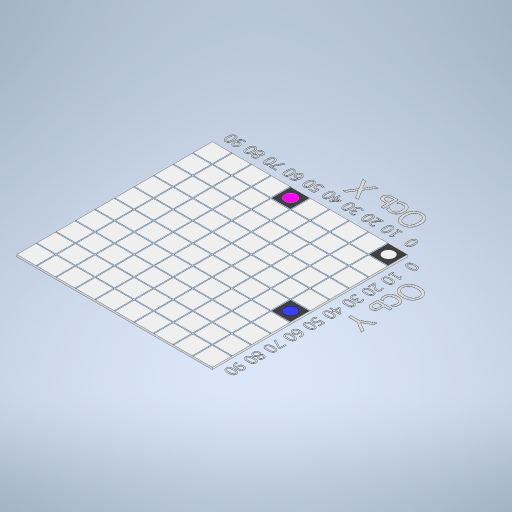
# Autodesk Inventor part: поле
Saved by Autodesk Inventor 2023.2 (Build 272271030, 271C)
## iProperties
Created: 2025-05-13
Part Number: поле
Material: Типовые
Document SubType Name: Modeling
Designer: e5470
Density: 1 g/cm^3
Appearance: По умолчанию
Author: e5470
Autodesk Inventor part; units mm, degrees
(part 1 of 3)
ref_plane "YZ Plane" through (0, 0, 0) normal (1, 0, 0) x (0, 1, 0)
ref_plane "XZ Plane" through (0, 0, 0) normal (0, 1, 0) x (-1, 0, 0)
ref_plane "XY Plane" through (0, 0, 0) normal (0, 0, 1) x (1, 0, 0)
sketch "Эскиз1" plane through (0, 0, 0) normal (0, 1, 0) x (-1, 0, 0)
  line L0 (-500, -500) -> (500, -500)
  line L1 (500, -500) -> (500, 500)
  line L2 (500, 500) -> (-500, 500)
  line L3 (-500, 500) -> (-500, -500)
  line L4 (-500, -500) -> (500, 500) construction
  line L5 (500, -500) -> (-500, 500) construction
  point P0 (0, 0)
  dimension "d0" = 1000
  dimension "d1" = 1000
  constraints: 12 end point, 2 midpoint, 2 parallel, 1 horizontal, 1 perpendicular
  measures "d0" distance of L2.end L1.end
  measures "d1" distance of L1.end L0.end
extrude "Выдавливание1" add sketch "Эскиз1" along normal blind 10
sketch "Эскиз2" plane through (0, 10, 0) normal (0, 1, 0) x (1, 0, 0)
  line L0 (500, -500) -> (500, 500) projected
  line L1 (-500, -2.5) -> (500, -2.5)
  line L2 (500, -2.5) -> (500, 2.5)
  line L3 (500, 2.5) -> (-500, 2.5)
  line L4 (-500, 2.5) -> (-500, -2.5)
  line L5 (-500, -2.5) -> (500, 2.5) construction
  line L6 (500, -2.5) -> (-500, 2.5) construction
  line L7 (-500, 97.5) -> (500, 97.5)
  line L8 (500, 97.5) -> (500, 102.5)
  line L9 (500, 102.5) -> (-500, 102.5)
  line L10 (-500, 102.5) -> (-500, 97.5)
  line L11 (-500, 97.5) -> (500, 102.5) construction
  line L12 (500, 97.5) -> (-500, 102.5) construction
  line L13 (-500, 197.5) -> (500, 197.5)
  line L14 (500, 197.5) -> (500, 202.5)
  line L15 (500, 202.5) -> (-500, 202.5)
  line L16 (-500, 202.5) -> (-500, 197.5)
  line L17 (-500, 197.5) -> (500, 202.5) construction
  line L18 (500, 197.5) -> (-500, 202.5) construction
  line L19 (-500, 297.5) -> (500, 297.5)
  line L20 (500, 297.5) -> (500, 302.5)
  line L21 (500, 302.5) -> (-500, 302.5)
  line L22 (-500, 302.5) -> (-500, 297.5)
  line L23 (-500, 297.5) -> (500, 302.5) construction
  line L24 (500, 297.5) -> (-500, 302.5) construction
  line L25 (-500, 397.5) -> (500, 397.5)
  line L26 (500, 397.5) -> (500, 402.5)
  line L27 (500, 402.5) -> (-500, 402.5)
  line L28 (-500, 402.5) -> (-500, 397.5)
  line L29 (-500, 397.5) -> (500, 402.5) construction
  line L30 (500, 397.5) -> (-500, 402.5) construction
  line L31 (-500, -102.5) -> (500, -102.5)
  line L32 (500, -102.5) -> (500, -97.5)
  line L33 (500, -97.5) -> (-500, -97.5)
  line L34 (-500, -97.5) -> (-500, -102.5)
  line L35 (-500, -102.5) -> (500, -97.5) construction
  line L36 (500, -102.5) -> (-500, -97.5) construction
  line L37 (-500, -2.5) -> (500, -2.5)
  line L38 (500, -2.5) -> (500, 2.5)
  line L39 (500, 2.5) -> (-500, 2.5)
  line L40 (-500, 2.5) -> (-500, -2.5)
  line L41 (-500, -2.5) -> (500, 2.5) construction
  line L42 (500, -2.5) -> (-500, 2.5) construction
  line L43 (-500, 97.5) -> (500, 97.5)
  line L44 (500, 97.5) -> (500, 102.5)
  line L45 (500, 102.5) -> (-500, 102.5)
  line L46 (-500, 102.5) -> (-500, 97.5)
  line L47 (-500, 97.5) -> (500, 102.5) construction
  line L48 (500, 97.5) -> (-500, 102.5) construction
  line L49 (-500, 197.5) -> (500, 197.5)
  line L50 (500, 197.5) -> (500, 202.5)
  line L51 (500, 202.5) -> (-500, 202.5)
  line L52 (-500, 202.5) -> (-500, 197.5)
  line L53 (-500, 197.5) -> (500, 202.5) construction
  line L54 (500, 197.5) -> (-500, 202.5) construction
  line L55 (-500, 297.5) -> (500, 297.5)
  line L56 (500, 297.5) -> (500, 302.5)
  line L57 (500, 302.5) -> (-500, 302.5)
  line L58 (-500, 302.5) -> (-500, 297.5)
  line L59 (-500, 297.5) -> (500, 302.5) construction
  line L60 (500, 297.5) -> (-500, 302.5) construction
  line L61 (-500, -202.5) -> (500, -202.5)
  line L62 (500, -202.5) -> (500, -197.5)
  line L63 (500, -197.5) -> (-500, -197.5)
  line L64 (-500, -197.5) -> (-500, -202.5)
  line L65 (-500, -202.5) -> (500, -197.5) construction
  line L66 (500, -202.5) -> (-500, -197.5) construction
  line L67 (-500, -102.5) -> (500, -102.5)
  line L68 (500, -102.5) -> (500, -97.5)
  line L69 (500, -97.5) -> (-500, -97.5)
  line L70 (-500, -97.5) -> (-500, -102.5)
  line L71 (-500, -102.5) -> (500, -97.5) construction
  line L72 (500, -102.5) -> (-500, -97.5) construction
  line L73 (-500, -2.5) -> (500, -2.5)
  line L74 (500, -2.5) -> (500, 2.5)
  line L75 (500, 2.5) -> (-500, 2.5)
  line L76 (-500, 2.5) -> (-500, -2.5)
  line L77 (-500, -2.5) -> (500, 2.5) construction
  line L78 (500, -2.5) -> (-500, 2.5) construction
  line L79 (-500, 97.5) -> (500, 97.5)
  line L80 (500, 97.5) -> (500, 102.5)
  line L81 (500, 102.5) -> (-500, 102.5)
  line L82 (-500, 102.5) -> (-500, 97.5)
  line L83 (-500, 97.5) -> (500, 102.5) construction
  line L84 (500, 97.5) -> (-500, 102.5) construction
  line L85 (-500, 197.5) -> (500, 197.5)
  line L86 (500, 197.5) -> (500, 202.5)
  line L87 (500, 202.5) -> (-500, 202.5)
  line L88 (-500, 202.5) -> (-500, 197.5)
  line L89 (-500, 197.5) -> (500, 202.5) construction
  line L90 (500, 197.5) -> (-500, 202.5) construction
  line L91 (-500, -302.5) -> (500, -302.5)
  line L92 (500, -302.5) -> (500, -297.5)
  line L93 (500, -297.5) -> (-500, -297.5)
  line L94 (-500, -297.5) -> (-500, -302.5)
  line L95 (-500, -302.5) -> (500, -297.5) construction
  line L96 (500, -302.5) -> (-500, -297.5) construction
  line L97 (-500, -202.5) -> (500, -202.5)
  line L98 (500, -202.5) -> (500, -197.5)
  line L99 (500, -197.5) -> (-500, -197.5)
  line L100 (-500, -197.5) -> (-500, -202.5)
  line L101 (-500, -202.5) -> (500, -197.5) construction
  line L102 (500, -202.5) -> (-500, -197.5) construction
  line L103 (-500, -102.5) -> (500, -102.5)
  line L104 (500, -102.5) -> (500, -97.5)
  line L105 (500, -97.5) -> (-500, -97.5)
  line L106 (-500, -97.5) -> (-500, -102.5)
  line L107 (-500, -102.5) -> (500, -97.5) construction
  line L108 (500, -102.5) -> (-500, -97.5) construction
  line L109 (-500, -2.5) -> (500, -2.5)
  line L110 (500, -2.5) -> (500, 2.5)
  line L111 (500, 2.5) -> (-500, 2.5)
  line L112 (-500, 2.5) -> (-500, -2.5)
  line L113 (-500, -2.5) -> (500, 2.5) construction
  line L114 (500, -2.5) -> (-500, 2.5) construction
  line L115 (-500, 97.5) -> (500, 97.5)
  line L116 (500, 97.5) -> (500, 102.5)
  line L117 (500, 102.5) -> (-500, 102.5)
  line L118 (-500, 102.5) -> (-500, 97.5)
  line L119 (-500, 97.5) -> (500, 102.5) construction
  line L120 (500, 97.5) -> (-500, 102.5) construction
  line L121 (-500, -402.5) -> (500, -402.5)
  line L122 (500, -402.5) -> (500, -397.5)
  line L123 (500, -397.5) -> (-500, -397.5)
  line L124 (-500, -397.5) -> (-500, -402.5)
  line L125 (-500, -402.5) -> (500, -397.5) construction
  line L126 (500, -402.5) -> (-500, -397.5) construction
  line L127 (-500, -302.5) -> (500, -302.5)
  line L128 (500, -302.5) -> (500, -297.5)
  line L129 (500, -297.5) -> (-500, -297.5)
  line L130 (-500, -297.5) -> (-500, -302.5)
  line L131 (-500, -302.5) -> (500, -297.5) construction
  line L132 (500, -302.5) -> (-500, -297.5) construction
  line L133 (-500, -202.5) -> (500, -202.5)
  line L134 (500, -202.5) -> (500, -197.5)
  line L135 (500, -197.5) -> (-500, -197.5)
  line L136 (-500, -197.5) -> (-500, -202.5)
  line L137 (-500, -202.5) -> (500, -197.5) construction
  line L138 (500, -202.5) -> (-500, -197.5) construction
  line L139 (-500, -102.5) -> (500, -102.5)
  line L140 (500, -102.5) -> (500, -97.5)
  line L141 (500, -97.5) -> (-500, -97.5)
  line L142 (-500, -97.5) -> (-500, -102.5)
  line L143 (-500, -102.5) -> (500, -97.5) construction
  line L144 (500, -102.5) -> (-500, -97.5) construction
  line L145 (-500, -2.5) -> (500, -2.5)
  line L146 (500, -2.5) -> (500, 2.5)
  line L147 (500, 2.5) -> (-500, 2.5)
  line L148 (-500, 2.5) -> (-500, -2.5)
  line L149 (-500, -2.5) -> (500, 2.5) construction
  line L150 (500, -2.5) -> (-500, 2.5) construction
  line L151 (2.5, 500) -> (-2.5, 500)
  line L152 (2.5, 500) -> (-2.5, 500)
  line L153 (2.5, 500) -> (-2.5, 500)
  line L154 (-97.5, -500) -> (-97.5, 500)
  line L155 (-97.5, 500) -> (-102.5, 500)
  line L156 (-102.5, 500) -> (-102.5, -500)
  line L157 (-102.5, -500) -> (-97.5, -500)
  line L158 (-97.5, -500) -> (-102.5, 500) construction
  line L159 (-97.5, 500) -> (-102.5, -500) construction
  line L160 (-97.5, -500) -> (-97.5, 500)
  line L161 (-97.5, -500) -> (-97.5, 500)
  line L162 (-97.5, -500) -> (-97.5, 500)
  line L163 (-97.5, -500) -> (-102.5, 500) construction
  line L164 (-97.5, 500) -> (-102.5, -500) construction
  line L165 (-97.5, -500) -> (-102.5, 500) construction
  line L166 (-97.5, 500) -> (-102.5, -500) construction
  line L167 (-97.5, -500) -> (-102.5, 500) construction
  line L168 (-97.5, 500) -> (-102.5, -500) construction
  line L169 (-102.5, 500) -> (-102.5, -500)
  line L170 (-102.5, 500) -> (-102.5, -500)
  line L171 (-102.5, 500) -> (-102.5, -500)
  line L172 (-102.5, -500) -> (-97.5, -500)
  line L173 (-102.5, -500) -> (-97.5, -500)
  line L174 (-102.5, -500) -> (-97.5, -500)
  line L175 (-297.5, -500) -> (-297.5, 500)
  line L176 (-297.5, -500) -> (-297.5, 500)
  line L177 (-297.5, 500) -> (-302.5, 500)
  line L178 (-302.5, 500) -> (-302.5, -500)
  line L179 (-297.5, -500) -> (-302.5, 500) construction
  line L180 (-302.5, 500) -> (-302.5, -500)
  line L181 (-297.5, -500) -> (-302.5, 500) construction
  line L182 (-297.5, 500) -> (-302.5, -500) construction
  line L183 (-397.5, -500) -> (-397.5, 500)
  line L184 (-402.5, 500) -> (-402.5, -500)
  line L185 (-397.5, 500) -> (-402.5, -500) construction
  line L186 (-397.5, -500) -> (-402.5, 500) construction
  line L187 (-397.5, 500) -> (-402.5, 500)
  line L188 (-297.5, 500) -> (-302.5, -500) construction
  line L189 (-302.5, -500) -> (-297.5, -500)
  line L190 (-302.5, -500) -> (-297.5, -500)
  line L191 (-402.5, -500) -> (-397.5, -500)
  line L192 (-197.5, -500) -> (-197.5, 500)
  line L193 (-197.5, 500) -> (-202.5, 500)
  line L194 (-202.5, 500) -> (-202.5, -500)
  line L195 (-202.5, -500) -> (-197.5, -500)
  line L196 (-197.5, -500) -> (-202.5, 500) construction
  line L197 (-197.5, 500) -> (-202.5, -500) construction
  line L198 (-202.5, 500) -> (-202.5, -500)
  line L199 (-202.5, 500) -> (-202.5, -500)
  line L200 (-197.5, 500) -> (-202.5, -500) construction
  line L201 (-197.5, 500) -> (-202.5, -500) construction
  line L202 (-197.5, -500) -> (-202.5, 500) construction
  line L203 (-197.5, -500) -> (-202.5, 500) construction
  line L204 (-197.5, 500) -> (-202.5, 500)
  line L205 (-197.5, 500) -> (-202.5, 500)
  line L206 (-197.5, -500) -> (-197.5, 500)
  line L207 (-197.5, -500) -> (-197.5, 500)
  line L208 (-202.5, -500) -> (-197.5, -500)
  line L209 (-202.5, -500) -> (-197.5, -500)
  line L210 (-97.5, 500) -> (-102.5, 500)
  line L211 (-97.5, 500) -> (-102.5, 500)
  line L212 (-97.5, 500) -> (-102.5, 500)
  line L213 (202.5, -500) -> (202.5, 500)
  line L214 (202.5, 500) -> (197.5, 500)
  line L215 (197.5, 500) -> (197.5, -500)
  line L216 (197.5, -500) -> (202.5, -500)
  line L217 (202.5, -500) -> (197.5, 500) construction
  line L218 (202.5, 500) -> (197.5, -500) construction
  line L219 (197.5, 500) -> (197.5, -500)
  line L220 (197.5, 500) -> (197.5, -500)
  line L221 (202.5, 500) -> (197.5, 500)
  line L222 (202.5, 500) -> (197.5, 500)
  line L223 (197.5, -500) -> (202.5, -500)
  line L224 (202.5, -500) -> (197.5, 500) construction
  line L225 (202.5, 500) -> (197.5, -500) construction
  line L226 (202.5, 500) -> (197.5, -500) construction
  line L227 (202.5, -500) -> (197.5, 500) construction
  line L228 (202.5, -500) -> (202.5, 500)
  line L229 (202.5, -500) -> (202.5, 500)
  line L230 (102.5, -500) -> (102.5, 500)
  line L231 (102.5, 500) -> (97.5, 500)
  line L232 (97.5, 500) -> (97.5, -500)
  line L233 (97.5, -500) -> (102.5, -500)
  line L234 (102.5, -500) -> (97.5, 500) construction
  line L235 (102.5, 500) -> (97.5, -500) construction
  line L236 (102.5, -500) -> (102.5, 500)
  line L237 (102.5, -500) -> (102.5, 500)
  line L238 (102.5, -500) -> (102.5, 500)
  line L239 (97.5, -500) -> (102.5, -500)
  line L240 (102.5, -500) -> (97.5, 500) construction
  line L241 (102.5, 500) -> (97.5, -500) construction
  line L242 (102.5, -500) -> (97.5, 500) construction
  line L243 (102.5, 500) -> (97.5, -500) construction
  line L244 (102.5, 500) -> (97.5, -500) construction
  line L245 (102.5, -500) -> (97.5, 500) construction
  line L246 (97.5, 500) -> (97.5, -500)
  line L247 (97.5, 500) -> (97.5, -500)
  line L248 (97.5, 500) -> (97.5, -500)
  line L249 (-297.5, 500) -> (-302.5, 500)
  line L250 (302.5, -500) -> (302.5, 500)
  line L251 (297.5, 500) -> (297.5, -500)
  line L252 (302.5, -500) -> (297.5, 500) construction
  line L253 (302.5, 500) -> (297.5, -500) construction
  line L254 (402.5, -500) -> (402.5, 500)
  line L255 (397.5, 500) -> (397.5, -500)
  line L256 (402.5, -500) -> (397.5, 500) construction
  line L257 (402.5, 500) -> (397.5, -500) construction
  line L258 (302.5, -500) -> (302.5, 500)
  line L259 (297.5, 500) -> (297.5, -500)
  line L260 (302.5, -500) -> (297.5, 500) construction
  line L261 (302.5, 500) -> (297.5, -500) construction
  line L262 (402.5, 500) -> (397.5, 500)
  line L263 (302.5, 500) -> (297.5, 500)
  line L264 (302.5, 500) -> (297.5, 500)
  line L265 (2.5, -500) -> (2.5, 500)
  line L266 (-2.5, 500) -> (-2.5, -500)
  line L267 (-2.5, -500) -> (2.5, -500)
  line L268 (2.5, -500) -> (-2.5, 500) construction
  line L269 (2.5, 500) -> (-2.5, -500) construction
  line L270 (-2.5, 500) -> (-2.5, -500)
  line L271 (-2.5, -500) -> (2.5, -500)
  line L272 (2.5, -500) -> (-2.5, 500) construction
  line L273 (2.5, 500) -> (-2.5, -500) construction
  line L274 (-2.5, 500) -> (-2.5, -500)
  line L275 (-2.5, -500) -> (2.5, -500)
  line L276 (2.5, -500) -> (-2.5, 500) construction
  line L277 (2.5, 500) -> (-2.5, -500) construction
  line L278 (2.5, -500) -> (-2.5, 500) construction
  line L279 (2.5, 500) -> (-2.5, -500) construction
  line L280 (2.5, -500) -> (-2.5, 500) construction
  line L281 (2.5, 500) -> (-2.5, -500) construction
  line L282 (-2.5, 500) -> (-2.5, -500)
  line L283 (-2.5, 500) -> (-2.5, -500)
  line L284 (2.5, -500) -> (2.5, 500)
  line L285 (2.5, -500) -> (2.5, 500)
  line L286 (2.5, -500) -> (2.5, 500)
  line L287 (2.5, -500) -> (2.5, 500)
  line L288 (102.5, 500) -> (97.5, 500)
  line L289 (102.5, 500) -> (97.5, 500)
  line L290 (102.5, 500) -> (97.5, 500)
  line L291 (97.5, -500) -> (102.5, -500)
  line L292 (-2.5, -500) -> (2.5, -500)
  line L293 (2.5, 500) -> (-2.5, 500)
  line L294 (2.5, 500) -> (-2.5, 500)
  line L295 (197.5, -500) -> (202.5, -500)
  line L296 (97.5, -500) -> (102.5, -500)
  line L297 (-2.5, -500) -> (2.5, -500)
  line L298 (297.5, -500) -> (302.5, -500)
  line L299 (297.5, -500) -> (302.5, -500)
  line L300 (397.5, -500) -> (402.5, -500)
  line L301 (-500, 2.5) -> (-500, -2.5)
  line L302 (-500, 2.5) -> (-500, -2.5)
  line L303 (-500, 2.5) -> (-500, -2.5)
  line L304 (500, -97.5) -> (-500, -97.5)
  line L305 (-500, -97.5) -> (-500, -102.5)
  line L306 (-500, -102.5) -> (500, -102.5)
  line L307 (500, -102.5) -> (500, -97.5)
  line L308 (500, -97.5) -> (-500, -102.5) construction
  line L309 (-500, -97.5) -> (500, -102.5) construction
  line L310 (500, -97.5) -> (-500, -97.5)
  line L311 (500, -97.5) -> (-500, -97.5)
  line L312 (500, -97.5) -> (-500, -97.5)
  line L313 (500, -97.5) -> (-500, -102.5) construction
  line L314 (-500, -97.5) -> (500, -102.5) construction
  line L315 (500, -97.5) -> (-500, -102.5) construction
  line L316 (-500, -97.5) -> (500, -102.5) construction
  line L317 (500, -97.5) -> (-500, -102.5) construction
  line L318 (-500, -97.5) -> (500, -102.5) construction
  line L319 (-500, -102.5) -> (500, -102.5)
  line L320 (-500, -102.5) -> (500, -102.5)
  line L321 (-500, -102.5) -> (500, -102.5)
  line L322 (500, -102.5) -> (500, -97.5)
  line L323 (500, -102.5) -> (500, -97.5)
  line L324 (500, -102.5) -> (500, -97.5)
  line L325 (500, -297.5) -> (-500, -297.5)
  line L326 (500, -297.5) -> (-500, -297.5)
  line L327 (-500, -297.5) -> (-500, -302.5)
  line L328 (-500, -302.5) -> (500, -302.5)
  line L329 (500, -297.5) -> (-500, -302.5) construction
  line L330 (-500, -302.5) -> (500, -302.5)
  line L331 (500, -297.5) -> (-500, -302.5) construction
  line L332 (-500, -297.5) -> (500, -302.5) construction
  line L333 (500, -397.5) -> (-500, -397.5)
  line L334 (-500, -402.5) -> (500, -402.5)
  line L335 (-500, -397.5) -> (500, -402.5) construction
  line L336 (500, -397.5) -> (-500, -402.5) construction
  line L337 (-500, -397.5) -> (-500, -402.5)
  line L338 (-500, -297.5) -> (500, -302.5) construction
  line L339 (500, -302.5) -> (500, -297.5)
  line L340 (500, -302.5) -> (500, -297.5)
  line L341 (500, -402.5) -> (500, -397.5)
  line L342 (500, -197.5) -> (-500, -197.5)
  line L343 (-500, -197.5) -> (-500, -202.5)
  line L344 (-500, -202.5) -> (500, -202.5)
  line L345 (500, -202.5) -> (500, -197.5)
  line L346 (500, -197.5) -> (-500, -202.5) construction
  line L347 (-500, -197.5) -> (500, -202.5) construction
  line L348 (-500, -202.5) -> (500, -202.5)
  line L349 (-500, -202.5) -> (500, -202.5)
  line L350 (-500, -197.5) -> (500, -202.5) construction
  line L351 (-500, -197.5) -> (500, -202.5) construction
  line L352 (500, -197.5) -> (-500, -202.5) construction
  line L353 (500, -197.5) -> (-500, -202.5) construction
  line L354 (-500, -197.5) -> (-500, -202.5)
  line L355 (-500, -197.5) -> (-500, -202.5)
  line L356 (500, -197.5) -> (-500, -197.5)
  line L357 (500, -197.5) -> (-500, -197.5)
  line L358 (500, -202.5) -> (500, -197.5)
  line L359 (500, -202.5) -> (500, -197.5)
  line L360 (-500, -97.5) -> (-500, -102.5)
  line L361 (-500, -97.5) -> (-500, -102.5)
  line L362 (-500, -97.5) -> (-500, -102.5)
  line L363 (500, 202.5) -> (-500, 202.5)
  line L364 (-500, 202.5) -> (-500, 197.5)
  line L365 (-500, 197.5) -> (500, 197.5)
  line L366 (500, 197.5) -> (500, 202.5)
  line L367 (500, 202.5) -> (-500, 197.5) construction
  line L368 (-500, 202.5) -> (500, 197.5) construction
  line L369 (-500, 197.5) -> (500, 197.5)
  line L370 (-500, 197.5) -> (500, 197.5)
  line L371 (-500, 202.5) -> (-500, 197.5)
  line L372 (-500, 202.5) -> (-500, 197.5)
  line L373 (500, 197.5) -> (500, 202.5)
  line L374 (500, 202.5) -> (-500, 197.5) construction
  line L375 (-500, 202.5) -> (500, 197.5) construction
  line L376 (-500, 202.5) -> (500, 197.5) construction
  line L377 (500, 202.5) -> (-500, 197.5) construction
  line L378 (500, 202.5) -> (-500, 202.5)
  line L379 (500, 202.5) -> (-500, 202.5)
  line L380 (500, 102.5) -> (-500, 102.5)
  line L381 (-500, 102.5) -> (-500, 97.5)
  line L382 (-500, 97.5) -> (500, 97.5)
  line L383 (500, 97.5) -> (500, 102.5)
  line L384 (500, 102.5) -> (-500, 97.5) construction
  line L385 (-500, 102.5) -> (500, 97.5) construction
  line L386 (500, 102.5) -> (-500, 102.5)
  line L387 (500, 102.5) -> (-500, 102.5)
  line L388 (500, 102.5) -> (-500, 102.5)
  line L389 (500, 97.5) -> (500, 102.5)
  line L390 (500, 102.5) -> (-500, 97.5) construction
  line L391 (-500, 102.5) -> (500, 97.5) construction
  line L392 (500, 102.5) -> (-500, 97.5) construction
  line L393 (-500, 102.5) -> (500, 97.5) construction
  line L394 (-500, 102.5) -> (500, 97.5) construction
  line L395 (500, 102.5) -> (-500, 97.5) construction
  line L396 (-500, 97.5) -> (500, 97.5)
  line L397 (-500, 97.5) -> (500, 97.5)
  line L398 (-500, 97.5) -> (500, 97.5)
  line L399 (-500, -297.5) -> (-500, -302.5)
  line L400 (500, 302.5) -> (-500, 302.5)
  line L401 (-500, 297.5) -> (500, 297.5)
  line L402 (500, 302.5) -> (-500, 297.5) construction
  line L403 (-500, 302.5) -> (500, 297.5) construction
  line L404 (500, 402.5) -> (-500, 402.5)
  line L405 (-500, 397.5) -> (500, 397.5)
  line L406 (500, 402.5) -> (-500, 397.5) construction
  line L407 (-500, 402.5) -> (500, 397.5) construction
  line L408 (500, 302.5) -> (-500, 302.5)
  line L409 (-500, 297.5) -> (500, 297.5)
  line L410 (500, 302.5) -> (-500, 297.5) construction
  line L411 (-500, 302.5) -> (500, 297.5) construction
  line L412 (-500, 402.5) -> (-500, 397.5)
  line L413 (-500, 302.5) -> (-500, 297.5)
  line L414 (-500, 302.5) -> (-500, 297.5)
  line L415 (500, 2.5) -> (-500, 2.5)
  line L416 (-500, -2.5) -> (500, -2.5)
  line L417 (500, -2.5) -> (500, 2.5)
  line L418 (500, 2.5) -> (-500, -2.5) construction
  line L419 (-500, 2.5) -> (500, -2.5) construction
  line L420 (-500, -2.5) -> (500, -2.5)
  line L421 (500, -2.5) -> (500, 2.5)
  line L422 (500, 2.5) -> (-500, -2.5) construction
  line L423 (-500, 2.5) -> (500, -2.5) construction
  line L424 (-500, -2.5) -> (500, -2.5)
  line L425 (500, -2.5) -> (500, 2.5)
  line L426 (500, 2.5) -> (-500, -2.5) construction
  line L427 (-500, 2.5) -> (500, -2.5) construction
  line L428 (500, 2.5) -> (-500, -2.5) construction
  line L429 (-500, 2.5) -> (500, -2.5) construction
  line L430 (500, 2.5) -> (-500, -2.5) construction
  line L431 (-500, 2.5) -> (500, -2.5) construction
  line L432 (-500, -2.5) -> (500, -2.5)
  line L433 (-500, -2.5) -> (500, -2.5)
  line L434 (500, 2.5) -> (-500, 2.5)
  line L435 (500, 2.5) -> (-500, 2.5)
  line L436 (500, 2.5) -> (-500, 2.5)
  line L437 (500, 2.5) -> (-500, 2.5)
  line L438 (-500, 102.5) -> (-500, 97.5)
  line L439 (-500, 102.5) -> (-500, 97.5)
  line L440 (-500, 102.5) -> (-500, 97.5)
  line L441 (500, 97.5) -> (500, 102.5)
  line L442 (500, -2.5) -> (500, 2.5)
  line L443 (-500, 2.5) -> (-500, -2.5)
  line L444 (-500, 2.5) -> (-500, -2.5)
  line L445 (500, 197.5) -> (500, 202.5)
  line L446 (500, 97.5) -> (500, 102.5)
  line L447 (500, -2.5) -> (500, 2.5)
  line L448 (500, 297.5) -> (500, 302.5)
  line L449 (500, 297.5) -> (500, 302.5)
  line L450 (500, 397.5) -> (500, 402.5)
  line L451 (-2.5, -500) -> (2.5, -500)
  line L452 (-2.5, -500) -> (2.5, -500)
  line L453 (-2.5, -500) -> (2.5, -500)
  line L454 (97.5, 500) -> (97.5, -500)
  line L455 (97.5, -500) -> (102.5, -500)
  line L456 (102.5, -500) -> (102.5, 500)
  line L457 (102.5, 500) -> (97.5, 500)
  line L458 (97.5, 500) -> (102.5, -500) construction
  line L459 (97.5, -500) -> (102.5, 500) construction
  line L460 (97.5, 500) -> (97.5, -500)
  line L461 (97.5, 500) -> (97.5, -500)
  line L462 (97.5, 500) -> (97.5, -500)
  line L463 (97.5, 500) -> (102.5, -500) construction
  line L464 (97.5, -500) -> (102.5, 500) construction
  line L465 (97.5, 500) -> (102.5, -500) construction
  line L466 (97.5, -500) -> (102.5, 500) construction
  line L467 (97.5, 500) -> (102.5, -500) construction
  line L468 (97.5, -500) -> (102.5, 500) construction
  line L469 (102.5, -500) -> (102.5, 500)
  line L470 (102.5, -500) -> (102.5, 500)
  line L471 (102.5, -500) -> (102.5, 500)
  line L472 (102.5, 500) -> (97.5, 500)
  line L473 (102.5, 500) -> (97.5, 500)
  line L474 (102.5, 500) -> (97.5, 500)
  line L475 (297.5, 500) -> (297.5, -500)
  line L476 (297.5, 500) -> (297.5, -500)
  line L477 (297.5, -500) -> (302.5, -500)
  line L478 (302.5, -500) -> (302.5, 500)
  line L479 (297.5, 500) -> (302.5, -500) construction
  line L480 (302.5, -500) -> (302.5, 500)
  line L481 (297.5, 500) -> (302.5, -500) construction
  line L482 (297.5, -500) -> (302.5, 500) construction
  line L483 (397.5, 500) -> (397.5, -500)
  line L484 (402.5, -500) -> (402.5, 500)
  line L485 (397.5, -500) -> (402.5, 500) construction
  line L486 (397.5, 500) -> (402.5, -500) construction
  line L487 (397.5, -500) -> (402.5, -500)
  line L488 (297.5, -500) -> (302.5, 500) construction
  line L489 (302.5, 500) -> (297.5, 500)
  line L490 (302.5, 500) -> (297.5, 500)
  line L491 (402.5, 500) -> (397.5, 500)
  line L492 (197.5, 500) -> (197.5, -500)
  line L493 (197.5, -500) -> (202.5, -500)
  line L494 (202.5, -500) -> (202.5, 500)
  line L495 (202.5, 500) -> (197.5, 500)
  line L496 (197.5, 500) -> (202.5, -500) construction
  line L497 (197.5, -500) -> (202.5, 500) construction
  line L498 (202.5, -500) -> (202.5, 500)
  line L499 (202.5, -500) -> (202.5, 500)
  line L500 (197.5, -500) -> (202.5, 500) construction
  line L501 (197.5, -500) -> (202.5, 500) construction
  line L502 (197.5, 500) -> (202.5, -500) construction
  line L503 (197.5, 500) -> (202.5, -500) construction
  line L504 (197.5, -500) -> (202.5, -500)
  line L505 (197.5, -500) -> (202.5, -500)
  line L506 (197.5, 500) -> (197.5, -500)
  line L507 (197.5, 500) -> (197.5, -500)
  line L508 (202.5, 500) -> (197.5, 500)
  line L509 (202.5, 500) -> (197.5, 500)
  line L510 (97.5, -500) -> (102.5, -500)
  line L511 (97.5, -500) -> (102.5, -500)
  line L512 (97.5, -500) -> (102.5, -500)
  line L513 (-202.5, 500) -> (-202.5, -500)
  line L514 (-202.5, -500) -> (-197.5, -500)
  line L515 (-197.5, -500) -> (-197.5, 500)
  line L516 (-197.5, 500) -> (-202.5, 500)
  line L517 (-202.5, 500) -> (-197.5, -500) construction
  line L518 (-202.5, -500) -> (-197.5, 500) construction
  line L519 (-197.5, -500) -> (-197.5, 500)
  line L520 (-197.5, -500) -> (-197.5, 500)
  line L521 (-202.5, -500) -> (-197.5, -500)
  line L522 (-202.5, -500) -> (-197.5, -500)
  line L523 (-197.5, 500) -> (-202.5, 500)
  line L524 (-202.5, 500) -> (-197.5, -500) construction
  line L525 (-202.5, -500) -> (-197.5, 500) construction
  line L526 (-202.5, -500) -> (-197.5, 500) construction
  line L527 (-202.5, 500) -> (-197.5, -500) construction
  line L528 (-202.5, 500) -> (-202.5, -500)
  line L529 (-202.5, 500) -> (-202.5, -500)
  line L530 (-102.5, 500) -> (-102.5, -500)
  line L531 (-102.5, -500) -> (-97.5, -500)
  line L532 (-97.5, -500) -> (-97.5, 500)
  line L533 (-97.5, 500) -> (-102.5, 500)
  line L534 (-102.5, 500) -> (-97.5, -500) construction
  line L535 (-102.5, -500) -> (-97.5, 500) construction
  line L536 (-102.5, 500) -> (-102.5, -500)
  line L537 (-102.5, 500) -> (-102.5, -500)
  line L538 (-102.5, 500) -> (-102.5, -500)
  line L539 (-97.5, 500) -> (-102.5, 500)
  line L540 (-102.5, 500) -> (-97.5, -500) construction
  line L541 (-102.5, -500) -> (-97.5, 500) construction
  line L542 (-102.5, 500) -> (-97.5, -500) construction
  line L543 (-102.5, -500) -> (-97.5, 500) construction
  line L544 (-102.5, -500) -> (-97.5, 500) construction
  line L545 (-102.5, 500) -> (-97.5, -500) construction
  line L546 (-97.5, -500) -> (-97.5, 500)
  line L547 (-97.5, -500) -> (-97.5, 500)
  line L548 (-97.5, -500) -> (-97.5, 500)
  line L549 (297.5, -500) -> (302.5, -500)
  line L550 (-302.5, 500) -> (-302.5, -500)
  line L551 (-297.5, -500) -> (-297.5, 500)
  line L552 (-302.5, 500) -> (-297.5, -500) construction
  line L553 (-302.5, -500) -> (-297.5, 500) construction
  line L554 (-402.5, 500) -> (-402.5, -500)
  line L555 (-397.5, -500) -> (-397.5, 500)
  line L556 (-402.5, 500) -> (-397.5, -500) construction
  line L557 (-402.5, -500) -> (-397.5, 500) construction
  line L558 (-302.5, 500) -> (-302.5, -500)
  line L559 (-297.5, -500) -> (-297.5, 500)
  line L560 (-302.5, 500) -> (-297.5, -500) construction
  line L561 (-302.5, -500) -> (-297.5, 500) construction
  line L562 (-402.5, -500) -> (-397.5, -500)
  line L563 (-302.5, -500) -> (-297.5, -500)
  line L564 (-302.5, -500) -> (-297.5, -500)
  line L565 (-2.5, 500) -> (-2.5, -500)
  line L566 (2.5, -500) -> (2.5, 500)
  line L567 (2.5, 500) -> (-2.5, 500)
  line L568 (-2.5, 500) -> (2.5, -500) construction
  line L569 (-2.5, -500) -> (2.5, 500) construction
  line L570 (2.5, -500) -> (2.5, 500)
  line L571 (2.5, 500) -> (-2.5, 500)
  line L572 (-2.5, 500) -> (2.5, -500) construction
  line L573 (-2.5, -500) -> (2.5, 500) construction
  line L574 (2.5, -500) -> (2.5, 500)
  line L575 (2.5, 500) -> (-2.5, 500)
  line L576 (-2.5, 500) -> (2.5, -500) construction
  line L577 (-2.5, -500) -> (2.5, 500) construction
  line L578 (-2.5, 500) -> (2.5, -500) construction
  line L579 (-2.5, -500) -> (2.5, 500) construction
  line L580 (-2.5, 500) -> (2.5, -500) construction
  line L581 (-2.5, -500) -> (2.5, 500) construction
  line L582 (2.5, -500) -> (2.5, 500)
  line L583 (2.5, -500) -> (2.5, 500)
  line L584 (-2.5, 500) -> (-2.5, -500)
  line L585 (-2.5, 500) -> (-2.5, -500)
  line L586 (-2.5, 500) -> (-2.5, -500)
  line L587 (-2.5, 500) -> (-2.5, -500)
  line L588 (-102.5, -500) -> (-97.5, -500)
  line L589 (-102.5, -500) -> (-97.5, -500)
  line L590 (-102.5, -500) -> (-97.5, -500)
  line L591 (-97.5, 500) -> (-102.5, 500)
  line L592 (2.5, 500) -> (-2.5, 500)
  line L593 (-2.5, -500) -> (2.5, -500)
  line L594 (-2.5, -500) -> (2.5, -500)
  line L595 (-197.5, 500) -> (-202.5, 500)
  line L596 (-97.5, 500) -> (-102.5, 500)
  line L597 (2.5, 500) -> (-2.5, 500)
  line L598 (-297.5, 500) -> (-302.5, 500)
  line L599 (-297.5, 500) -> (-302.5, 500)
  line L600 (-397.5, 500) -> (-402.5, 500)
  point P0 (0, 0)
  point P1 (0, 100)
  point P2 (0, 200)
  point P3 (0, 300)
  point P4 (0, 400)
  point P5 (0, -100)
  point P6 (0, 0)
  point P7 (0, 100)
  point P8 (0, 200)
  point P9 (0, 300)
  point P10 (0, -200)
  point P11 (0, -100)
  point P12 (0, 0)
  point P13 (0, 100)
  point P14 (0, 200)
  point P15 (0, -300)
  point P16 (0, -200)
  point P17 (0, -100)
  point P18 (0, 0)
  point P19 (0, 100)
  point P20 (0, -400)
  point P21 (0, -300)
  point P22 (0, -200)
  point P23 (0, -100)
  point P24 (0, 0)
  point P25 (-100, 0)
  point P26 (-100, 0)
  point P27 (-100, 0)
  point P28 (-100, 0)
  point P29 (-300, 0)
  point P30 (-300, 0)
  point P31 (-400, 0)
  point P32 (-200, 0)
  point P33 (-200, 0)
  point P34 (-200, 0)
  point P35 (200, 0)
  point P36 (200, 0)
  point P37 (200, 0)
  point P38 (100, 0)
  point P39 (100, 0)
  point P40 (100, 0)
  point P41 (100, 0)
  point P42 (300, 0)
  point P43 (400, 0)
  point P44 (300, 0)
  point P45 (0, 0)
  point P46 (0, 0)
  point P47 (0, 0)
  point P48 (0, 0)
  point P49 (0, 0)
  point P50 (0, -100)
  point P51 (0, -100)
  point P52 (0, -100)
  point P53 (0, -100)
  point P54 (0, -300)
  point P55 (0, -300)
  point P56 (0, -400)
  point P57 (0, -200)
  point P58 (0, -200)
  point P59 (0, -200)
  point P60 (0, 200)
  point P61 (0, 200)
  point P62 (0, 200)
  point P63 (0, 100)
  point P64 (0, 100)
  point P65 (0, 100)
  point P66 (0, 100)
  point P67 (0, 300)
  point P68 (0, 400)
  point P69 (0, 300)
  point P70 (0, 0)
  point P71 (0, 0)
  point P72 (0, 0)
  point P73 (0, 0)
  point P74 (0, 0)
  point P75 (100, 0)
  point P76 (100, 0)
  point P77 (100, 0)
  point P78 (100, 0)
  point P79 (300, 0)
  point P80 (300, 0)
  point P81 (400, 0)
  point P82 (200, 0)
  point P83 (200, 0)
  point P84 (200, 0)
  point P85 (-200, 0)
  point P86 (-200, 0)
  point P87 (-200, 0)
  point P88 (-100, 0)
  point P89 (-100, 0)
  point P90 (-100, 0)
  point P91 (-100, 0)
  point P92 (-300, 0)
  point P93 (-400, 0)
  point P94 (-300, 0)
  point P95 (0, 0)
  point P96 (0, 0)
  point P97 (0, 0)
  point P98 (0, 0)
  point P99 (0, 0)
  point P100 (197.5, -302.5)
  point P101 (197.5, -397.5)
  point P102 (102.5, -397.5)
  point P103 (102.5, -302.5)
  point P104 (197.5, -297.5)
  point P105 (102.5, -297.5)
  point P106 (102.5, -202.5)
  point P107 (197.5, -202.5)
  point P108 (97.5, -102.5)
  point P109 (97.5, -197.5)
  point P110 (2.5, -197.5)
  point P111 (2.5, -102.5)
  point P112 (97.5, -97.5)
  point P113 (2.5, -97.5)
  point P114 (2.5, -2.5)
  point P115 (97.5, -2.5)
  point P116 (-2.5, 97.5)
  point P117 (-2.5, 2.5)
  point P118 (-97.5, 2.5)
  point P119 (-97.5, 97.5)
  point P120 (-2.5, 102.5)
  point P121 (-97.5, 102.5)
  point P122 (-97.5, 197.5)
  point P123 (-2.5, 197.5)
  point P124 (-97.5, 402.5)
  point P125 (-102.5, 402.5)
  point P126 (-197.5, 402.5)
  point P127 (-202.5, 402.5)
  point P128 (-297.5, 402.5)
  point P129 (-302.5, 402.5)
  point P130 (-397.5, 402.5)
  point P131 (-402.5, 402.5)
  point P132 (-402.5, 397.5)
  point P133 (-402.5, 302.5)
  point P134 (-402.5, 297.5)
  point P135 (-402.5, 202.5)
  point P136 (-402.5, 197.5)
  point P137 (-402.5, 102.5)
  point P138 (-402.5, 97.5)
  point P139 (-402.5, 2.5)
  point P140 (-402.5, -2.5)
  point P141 (-402.5, -97.5)
  point P142 (-402.5, -102.5)
  point P143 (-402.5, -197.5)
  point P144 (-402.5, -202.5)
  point P145 (-402.5, -297.5)
  point P146 (-402.5, -302.5)
  point P147 (-402.5, -397.5)
  point P148 (-402.5, -402.5)
  point P149 (-397.5, -402.5)
  point P150 (-302.5, -402.5)
  point P151 (-297.5, -402.5)
  point P152 (-202.5, -402.5)
  point P153 (-197.5, -402.5)
  point P154 (-102.5, -402.5)
  point P155 (-97.5, -402.5)
  point P156 (-2.5, -402.5)
  point P157 (2.5, -402.5)
  point P158 (97.5, -402.5)
  point P159 (102.5, -402.5)
  point P160 (197.5, -402.5)
  point P161 (202.5, -402.5)
  point P162 (297.5, -402.5)
  point P163 (302.5, -402.5)
  point P164 (397.5, -402.5)
  point P165 (402.5, -402.5)
  point P166 (402.5, -397.5)
  point P167 (402.5, -302.5)
  point P168 (402.5, -297.5)
  point P169 (402.5, -202.5)
  point P170 (402.5, -197.5)
  point P171 (402.5, -102.5)
  point P172 (402.5, -97.5)
  point P173 (402.5, -2.5)
  point P174 (402.5, 2.5)
  point P175 (402.5, 97.5)
  point P176 (402.5, 102.5)
  point P177 (402.5, 197.5)
  point P178 (402.5, 202.5)
  point P179 (402.5, 297.5)
  point P180 (402.5, 302.5)
  point P181 (402.5, 397.5)
  point P182 (402.5, 402.5)
  point P183 (397.5, 402.5)
  point P184 (302.5, 402.5)
  point P185 (297.5, 402.5)
  point P186 (202.5, 402.5)
  point P187 (197.5, 402.5)
  point P188 (102.5, 402.5)
  point P189 (97.5, 402.5)
  point P190 (2.5, 402.5)
  point P191 (-2.5, 402.5)
  point P192 (-97.5, 397.5)
  point P193 (-2.5, 397.5)
  point P194 (-2.5, 302.5)
  point P195 (-97.5, 302.5)
  point P196 (-97.5, 297.5)
  point P197 (-2.5, 297.5)
  point P198 (-2.5, 202.5)
  point P199 (-97.5, 202.5)
  dimension "d4" = 5
  dimension "d7" = 100
  dimension "d10" = 100
  dimension "d15" = 360
  constraints: 1166 end point, 17 vertical, 10 perpendicular, 2 coincident, 2 collinear, 2 midpoint, 1 horizontal, 1 parallel, 1 point on line, 1388 other
  measures "d4" distance of L2.end L2.start
  measures "d7" distance of L4.end L10.end
  measures "d10" distance of L4.end L34.end
extrude "Выдавливание2" add sketch "Эскиз2" along normal blind 0.1 separate body contours L121 L254 L123 L0 | L254 L300 L255 L121 | L121 L255 L123 L254 | L91 L254 L93 L0 | L123 L255 L91 L254 | L121 L250 L123 L255 | L91 L255 L93 L254 | L250 L298 L251 L121 | L121 L251 L123 L250 | L61 L254 L63 L0 | L93 L255 L61 L254 | L91 L250 L93 L255 | L123 L251 L91 L250 | L121 L213 L123 L251 | L61 L255 L63 L254 | L91 L251 L93 L250 | L213 L216 L215 L121 | L121 L215 L123 L213 | L31 L254 L33 L0 | L63 L255 L31 L254 | L61 L250 L63 L255 | L93 L251 L61 L250 | L91 L213 L93 L251 | L123 L215 L91 L213 | L121 L230 L123 L215 | L31 L255 L33 L254 | L61 L251 L63 L250 | L91 L215 L93 L213 | L230 L233 L232 L121 | L121 L232 L123 L230 | L1 L254 L3 L0 | L33 L255 L1 L254 | L31 L250 L33 L255 | L63 L251 L31 L250 | L61 L213 L63 L251 | L93 L215 L61 L213 | L91 L230 L93 L215 | L123 L232 L91 L230 | L121 L265 L123 L232 | L1 L255 L3 L254 | L31 L251 L33 L250 | L61 L215 L63 L213 | L91 L232 L93 L230 | L265 L267 L266 L121 | L121 L266 L123 L265 | L7 L254 L9 L0 | L3 L255 L7 L254 | L1 L250 L3 L255 | L33 L251 L1 L250 | L31 L213 L33 L251 | L63 L215 L31 L213 | L61 L230 L63 L215 | L93 L232 L61 L230 | L91 L265 L93 L232 | L123 L266 L91 L265 | L121 L154 L123 L266 | L7 L255 L9 L254 | L1 L251 L3 L250 | L31 L215 L33 L213 | L61 L232 L63 L230 | L91 L266 L93 L265 | L154 L157 L156 L121 | L121 L156 L123 L154 | L13 L254 L15 L0 | L9 L255 L13 L254 | L7 L250 L9 L255 | L3 L251 L7 L250 | L1 L213 L3 L251 | L33 L215 L1 L213 | L31 L230 L33 L215 | L63 L232 L31 L230 | L61 L265 L63 L232 | L93 L266 L61 L265 | L91 L154 L93 L266 | L123 L156 L91 L154 | L121 L192 L123 L156 | L13 L255 L15 L254 | L7 L251 L9 L250 | L1 L215 L3 L213 | L31 L232 L33 L230 | L61 L266 L63 L265 | L91 L156 L93 L154 | L192 L195 L194 L121 | L121 L194 L123 L192 | L19 L254 L21 L0 | L15 L255 L19 L254 | L13 L250 L15 L255 | L9 L251 L13 L250 | L7 L213 L9 L251 | L3 L215 L7 L213 | L1 L230 L3 L215 | L33 L232 L1 L230 | L31 L265 L33 L232 | L63 L266 L31 L265 | L61 L154 L63 L266 | L93 L156 L61 L154 | L91 L192 L93 L156 | L123 L194 L91 L192 | L121 L175 L123 L194 | L19 L255 L21 L254 | L13 L251 L15 L250 | L7 L215 L9 L213 | L1 L232 L3 L230 | L31 L266 L33 L265 | L61 L156 L63 L154 | L91 L194 L93 L192 | L175 L189 L178 L121 | L121 L178 L123 L175 | L25 L254 L27 L0 | L21 L255 L25 L254 | L19 L250 L21 L255 | L15 L251 L19 L250 | L13 L213 L15 L251 | L9 L215 L13 L213 | L7 L230 L9 L215 | L3 L232 L7 L230 | L1 L265 L3 L232 | L33 L266 L1 L265 | L31 L154 L33 L266 | L63 L156 L31 L154 | L61 L192 L63 L156 | L93 L194 L61 L192 | L91 L175 L93 L194 | L123 L178 L91 L175 | L121 L183 L123 L178 | L25 L255 L27 L254 | L19 L251 L21 L250 | L13 L215 L15 L213 | L7 L232 L9 L230 | L1 L266 L3 L265 | L31 L156 L33 L154 | L61 L194 L63 L192 | L91 L178 L93 L175 | L183 L191 L184 L121 | L121 L184 L123 L183 | L27 L255 L262 L254 | L25 L250 L27 L255 | L21 L251 L25 L250 | L19 L213 L21 L251 | L15 L215 L19 L213 | L13 L230 L15 L215 | L9 L232 L13 L230 | L7 L265 L9 L232 | L3 L266 L7 L265 | L1 L154 L3 L266 | L33 L156 L1 L154 | L31 L192 L33 L156 | L63 L194 L31 L192 | L61 L175 L63 L194 | L93 L178 L61 L175 | L91 L183 L93 L178 | L123 L184 L91 L183 | L121 L124 L123 L184 | L25 L251 L27 L250 | L19 L215 L21 L213 | L13 L232 L15 L230 | L7 L266 L9 L265 | L1 L156 L3 L154 | L31 L194 L33 L192 | L61 L178 L63 L175 | L91 L184 L93 L183 | L27 L251 L263 L250 | L25 L213 L27 L251 | L21 L215 L25 L213 | L19 L230 L21 L215 | L15 L232 L19 L230 | L13 L265 L15 L232 | L9 L266 L13 L265 | L7 L154 L9 L266 | L3 L156 L7 L154 | L1 L192 L3 L156 | L33 L194 L1 L192 | L31 L175 L33 L194 | L63 L178 L31 L175 | L61 L183 L63 L178 | L93 L184 L61 L183 | L91 L94 L93 L184 | L25 L215 L27 L213 | L19 L232 L21 L230 | L13 L266 L15 L265 | L7 L156 L9 L154 | L1 L194 L3 L192 | L31 L178 L33 L175 | L61 L184 L63 L183 | L27 L215 L214 L213 | L25 L230 L27 L215 | L21 L232 L25 L230 | L19 L265 L21 L232 | L15 L266 L19 L265 | L13 L154 L15 L266 | L9 L156 L13 L154 | L7 L192 L9 L156 | L3 L194 L7 L192 | L1 L175 L3 L194 | L33 L178 L1 L175 | L31 L183 L33 L178 | L63 L184 L31 L183 | L61 L64 L63 L184 | L25 L232 L27 L230 | L19 L266 L21 L265 | L13 L156 L15 L154 | L7 L194 L9 L192 | L1 L178 L3 L175 | L31 L184 L33 L183 | L27 L232 L231 L230 | L25 L265 L27 L232 | L21 L266 L25 L265 | L19 L154 L21 L266 | L15 L156 L19 L154 | L13 L192 L15 L156 | L9 L194 L13 L192 | L7 L175 L9 L194 | L3 L178 L7 L175 | L1 L183 L3 L178 | L33 L184 L1 L183 | L31 L34 L33 L184 | L25 L266 L27 L265 | L19 L156 L21 L154 | L13 L194 L15 L192 | L7 L178 L9 L175 | L1 L184 L3 L183 | L27 L266 L151 L265 | L25 L154 L27 L266 | L21 L156 L25 L154 | L19 L192 L21 L156 | L15 L194 L19 L192 | L13 L175 L15 L194 | L9 L178 L13 L175 | L7 L183 L9 L178 | L3 L184 L7 L183 | L1 L4 L3 L184 | L25 L156 L27 L154 | L19 L194 L21 L192 | L13 L178 L15 L175 | L7 L184 L9 L183 | L27 L156 L155 L154 | L25 L192 L27 L156 | L21 L194 L25 L192 | L19 L175 L21 L194 | L15 L178 L19 L175 | L13 L183 L15 L178 | L9 L184 L13 L183 | L7 L10 L9 L184 | L25 L194 L27 L192 | L19 L178 L21 L175 | L13 L184 L15 L183 | L27 L194 L193 L192 | L25 L175 L27 L194 | L21 L178 L25 L175 | L19 L183 L21 L178 | L15 L184 L19 L183 | L13 L16 L15 L184 | L25 L178 L27 L175 | L19 L184 L21 L183 | L27 L178 L177 L175 | L25 L183 L27 L178 | L21 L184 L25 L183 | L19 L22 L21 L184 | L25 L184 L27 L183 | L27 L184 L187 L183 | L25 L28 L27 L184